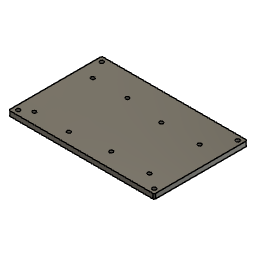
monitor_route_bar (Autodesk Fusion 360 design; units mm, degrees)
Autodesk Fusion 360 part; units mm, degrees
note: some values were not read from the file. Set by a fixed rule: the direction of a hole.
sketch "スケッチ1" plane through (0, 0, 0) normal (0, 1, 0) x (1, 0, 0)
  line L0 (57, 35) -> (-57, 35)
  line L1 (-57, 35) -> (-57, -35)
  line L2 (-57, -35) -> (57, -35)
  line L3 (57, -35) -> (57, 35)
  line L4 (57, 35) -> (-57, -35) construction
  line L5 (-57, 35) -> (57, -35) construction
  line L6 (61, 39) -> (-61, 39)
  line L7 (-61, 39) -> (-61, -39)
  line L8 (-61, -39) -> (61, -39)
  line L9 (61, -39) -> (61, 39)
  line L10 (61, 39) -> (-61, -39) construction
  line L11 (-61, 39) -> (61, -39) construction
  dimension "d9" = 114
  dimension "d10" = 70
  dimension "d11" = 78
  dimension "d12" = 122
  constraint horizontal L0
  constraint perpendicular L0 L1
  constraint parallel L0 L2
  constraint parallel L1 L3
  constraint coincident L4 origin
  constraint coincident L5 origin
  constraint horizontal L6
  constraint perpendicular L6 L7
  constraint parallel L6 L8
  constraint parallel L7 L9
  constraint coincident L10 origin
  constraint coincident L11 origin
  measures "d9" distance of L0.start L0.end
  measures "d10" distance of L0.end L1.end
  measures "d11" distance of L6.start L8.end
  measures "d12" distance of L7.end L8.end
extrude "押し出し1" add sketch "スケッチ1" along normal blind 4 contours L0 L1 L2 L3 | L6 L7 L8 L9
hole "穴1" at (-57, 0, -35) at (-57, 0, 35) at (57, 0, 35) at (57, 0, -35) direction (0, 1, 0) diameter 3.2 end through all
sketch "スケッチ2" plane through (0, 4, 0) normal (0, 1, 0) x (-1, 0, 0)
  circle A0 centre (-57, 35) radius 1.6
  circle A1 centre (57, -35) radius 1.6
  circle A2 centre (57, 35) radius 1.6
  circle A3 centre (-57, -35) radius 1.6
  line L0 (-61, 39) -> (-61, -39)
  line L1 (-61, -39) -> (61, -39)
  line L2 (61, -39) -> (61, 39)
  line L3 (61, 39) -> (-61, 39)
  line L4 (49, -19.5) -> (20, -19.5)
  line L5 (20, -19.5) -> (20, 29.5)
  line L6 (20, 29.5) -> (49, 29.5)
  line L7 (49, 29.5) -> (49, -19.5)
  line L8 (-12, -16) -> (-12, 26)
  line L9 (-44, -16) -> (-44, 26)
  point P0 (-12, 5)
  point P1 (-44, 5)
  point P2 (20, 5)
  dimension "d13" = 29
  dimension "d14" = 49
  dimension "d15" = 12
  dimension "d16" = 42
  dimension "d17" = 42
  dimension "d18" = 32
  dimension "d19" = 17
  dimension "d25" = 5
  constraint horizontal L4
  constraint vertical L5
  constraint horizontal L6
  constraint vertical L7
  constraint vertical L8
  constraint vertical L9
  constraint midpoint L8 P0
  constraint midpoint L9 P1
  constraint midpoint L5 P2
  constraint horizontal P0 P2
  constraint horizontal P0 P1
  measures "d13" distance of L4.start L4.end
  measures "d14" distance of L4.start L6.end
  measures "d15" distance of L2 L7
  measures "d16" distance of L9.start L9.end
  measures "d17" distance of L8.start L8.end
  measures "d18" distance of L5 L8
  measures "d19" distance of L0 L9
  measures "d25" vertical distance of origin P1
hole "穴2" at (-49, 4, -19.5) at (-49, 4, 29.5) at (-20, 4, 29.5) at (-20, 4, -19.5) at (44, 4, -16) at (44, 4, 26) at (12, 4, -16) at (12, 4, 26) direction (0, -1, 0) diameter 3 end through all
fillet "フィレット1" radius 1 4 edges at (61, 2, 39) (61, 2, -39) (-61, 2, 39) (-61, 2, -39)
